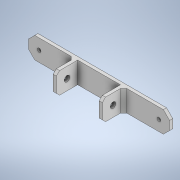
# Autodesk Inventor part: soporte router
Saved by Autodesk Inventor 2022 (Build 260153000, 153)
## iProperties
Created: 2022-02-18
Part Number: soporte router
Material: Generic
Document SubType Name: Modeling
Designer: juanp
Density: 1 g/cm^3
Appearance: Default
Author: juanp
Autodesk Inventor part; units mm, degrees
ref_plane "YZ Plane" through (0, 0, 0) normal (1, 0, 0) x (0, 1, 0)
ref_plane "XZ Plane" through (0, 0, 0) normal (0, 1, 0) x (-1, 0, 0)
ref_plane "XY Plane" through (0, 0, 0) normal (0, 0, 1) x (1, 0, 0)
sketch "Sketch1" plane through (0, 0, 0) normal (0, 0, 1) x (1, 0, 0)
  line L0 (-56.25, 0) -> (56.25, 0) construction
  circle A0 centre (-56.25, 0) radius 1.75
  circle A1 centre (56.25, 0) radius 1.75
  line L1 (-56.25, 0) -> (56.25, 0) construction
  line L2 (-56.25, 10) -> (56.25, 10)
  line L3 (56.25, -10) -> (-56.25, -10)
  arc A2 (-56.25, 10) -> (-56.25, -10) centre (-56.25, 0) ccw
  arc A3 (56.25, -10) -> (56.25, 10) centre (56.25, 0) ccw
  line L4 (-23.1, 10) -> (-20.1, 10)
  line L5 (-20.1, 10) -> (-20.1, -10)
  line L6 (-20.1, -10) -> (-23.1, -10)
  line L7 (-23.1, -10) -> (-23.1, 10)
  line L8 (20.1, 10) -> (23.1, 10)
  line L9 (23.1, 10) -> (23.1, -10)
  line L10 (23.1, -10) -> (20.1, -10)
  line L11 (20.1, -10) -> (20.1, 10)
  line L12 (-20.1, 0) -> (20.1, 0) construction
  line L13 (0, 0) -> (0, 10) construction
  line L14 (-66.25, -4.1421) -> (-66.25, 4.1421)
  line L15 (-66.25, 4.1421) -> (-60.3921, 10)
  line L16 (-60.3921, 10) -> (-52.1079, 10)
  line L17 (-52.1079, 10) -> (-46.25, 4.1421)
  line L18 (-46.25, 4.1421) -> (-46.25, -4.1421)
  line L19 (-46.25, -4.1421) -> (-52.1079, -10)
  line L20 (-52.1079, -10) -> (-60.3921, -10)
  line L21 (-60.3921, -10) -> (-66.25, -4.1421)
  line L22 (60.3921, -10) -> (52.1079, -10)
  line L23 (52.1079, -10) -> (46.25, -4.1421)
  line L24 (46.25, -4.1421) -> (46.25, 4.1421)
  line L25 (46.25, 4.1421) -> (52.1079, 10)
  line L26 (52.1079, 10) -> (60.3921, 10)
  line L27 (60.3921, 10) -> (66.25, 4.1421)
  line L28 (66.25, 4.1421) -> (66.25, -4.1421)
  line L29 (66.25, -4.1421) -> (60.3921, -10)
  point P0 (63.3211, -7.0711)
  point P1 (66.25, 0)
  point P2 (56.25, -10)
  point P3 (63.3211, 7.0711)
  point P4 (56.25, 10)
  point P5 (-63.3211, -7.0711)
  point P6 (-66.25, 0)
  point P7 (-63.3211, 7.0711)
  dimension "d0" = 112.5
  dimension "d1" = 3.5
  dimension "d4" = 10
  dimension "d5" = 3
  dimension "d6" = 3
  dimension "d7" = 40.2
  constraints: 62 end point, 6 horizontal, 6 midpoint, 5 coincident, 5 parallel, 4 centre point, 4 perpendicular, 4 point on circle, 4 tangent, 3 collinear, 3 point on line, 1 equal length, 1 equal radius, 34 other
  measures "d0" distance of L0.start L0.end
  measures "d1" diameter of A0
  measures "d4" radius of A2
  measures "d5" distance between parallel lines of L5 L7
  measures "d6" distance between parallel lines of L11 L9
  measures "d7" distance between parallel lines of L11 L5
extrude "Extrusion1" add sketch "Sketch1" along normal blind 3
extrude "Extrusion2" add sketch "Sketch1" along normal blind 23 contours L2 L5 L3 L7 | L2 L9 L3 L11
sketch "Sketch2" plane through (23.1, -10, 3) normal (1, 0, 0) x (0, 0, -1)
  line L0 (0, 0) -> (-20, 20) construction
  circle A0 centre (-10, 10) radius 2.65
  point P0 (3, 10)
  dimension "d12" = 5.3
  constraints: 2 end point, 1 centre point, 1 coincident, 1 midpoint
  measures "d12" diameter of A0
extrude "Extrusion3" cut sketch "Sketch2" against normal through all
chamfer "Chamfer1" distance 3 angle 45 6 edges at (23.1, 0, 3) (-23.1, 0, 3) (21.6, 10, 23) (21.6, -10, 23) (-21.6, -10, 23) (-21.6, 10, 23)
body "Solid1"
